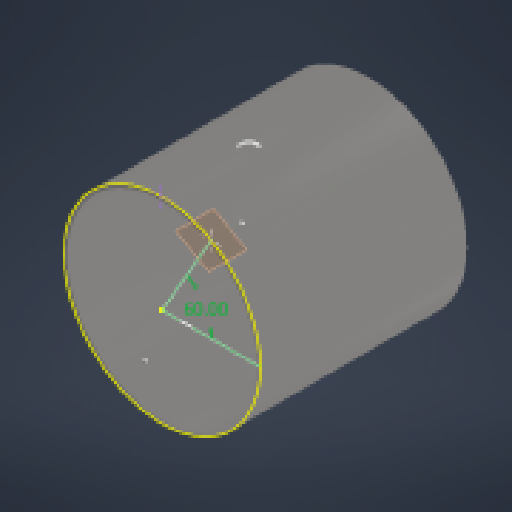
# Autodesk Inventor part: Electromagnetic cover body
Saved by Autodesk Inventor 2026.3 (Build 303398000, 398)
## iProperties
Created: 2026-08-03
Part Number: Electromagnetic cover body
Material: Generic
Document SubType Name: Sheet Metal
Designer: matot
Density: 1 g/cm^3
Sheet Metal Rule: Default_mm
Appearance: Default
Author: matot
Autodesk Inventor part; units mm, degrees
ref_plane "YZ Plane" through (0, 0, 0) normal (1, 0, 0) x (0, 1, 0)
ref_plane "XZ Plane" through (0, 0, 0) normal (0, 1, 0) x (-1, 0, 0)
sketch "Sketch1" plane through (0, 0, 0) normal (0, 0, 1) x (1, 0, 0)
  circle A0 centre (0, 0) radius 57
  circle A1 centre (0, 0) radius 55
  dimension "d0" = 114
  dimension "d1" = 110
  constraints: 2 centre point, 2 coincident
  measures "d0" diameter of A0
  measures "d1" diameter of A1
extrude "Extrusion1" add sketch "Sketch1" along normal blind 120
sketch "Sketch2" plane through (0, 0, 120) normal (0, 0, 1) x (1, 0, 0)
  circle A0 centre (0, 0) radius 57 projected
  point P0 (0, 57)
  constraints: 1 vertical alignment, 1 other
ref_plane "Work Plane1" through (0, 57, 120) normal (0, 1, 0) x (-1, 0, 0)
sketch "Sketch3" plane through (0, 57, 120) normal (0, 1, 0) x (-1, 0, 0)
  line L0 (57, 0) -> (-57, 0) projected
  point P0 (0, -120)
  point P1 (0, -50)
  dimension "d4" = 50
  measures "d4" distance from line of L0 point (0, -50)
hole "Hole1" at (0, 57, 70) direction (0, -1, 0) diameter 10 depth 20 tip angle 118
sketch "Sketch6" plane through (0, 0, 120) normal (0, 0, 1) x (1, 0, 0)
  circle A0 centre (0, 0) radius 57 projected
  point P0 (0, 57)
  constraints: 1 vertical alignment, 1 other
sketch "Sketch11" plane through (0, 0, 120) normal (0, 0, 1) x (1, 0, 0)
  circle A0 centre (0, 0) radius 57 projected
  line L0 (28.5, 49.3634) -> (0, 0)
  line L1 (57, 0) -> (0, 0)
  dimension "d47" = 60
  constraints: 4 end point, 2 point on circle, 1 horizontal
ref_plane "Work Plane7" through (28.5, 49.3634, 120) normal (0.5, 0.8660254, 0) x (-0.8660254, 0.5, 0)
sketch "Sketch12" plane through (28.5, 49.3634, 120) normal (0.5, 0.8660254, 0) x (-0.8660254, 0.5, 0)
  line L0 (57, 0) -> (-57, 0) projected
  point P0 (0, -120)
  point P1 (0, -17.607)
  dimension "d48" = 17.607
  measures "d48" distance from line of point (0, -17.607) L0
hole "Hole6" at (28.5, 49.3634, 102.393) direction (-0.5, -0.8660254, 0) diameter 2 end through all
equation "\"d54\" = Thickness"
equation "\"BendRadius\" = Thickness"
equation "\"BendReliefWidth\" = Thickness"
equation "\"BendReliefDepth\" = 0.5 * Thickness"
equation "\"CornerReliefSize\" = 4 * Thickness"
equation "\"MinimumRemnant\" = 2 * Thickness"
equation "\"TransitionRadius\" = BendRadius"
equation "\"JacobiRadiusSize\" = BendRadius"
equation "\"GapSize\" = Thickness"
equation "\"Thickness\" = 0.5"
body "Solid1"
